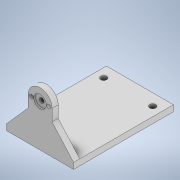
# Autodesk Inventor part: encoder_mount
Saved by Autodesk Inventor 2022 (Build 260153000, 153)
## iProperties
Created: 2021-12-21
Part Number: encoder_mount
Material: Generic
Document SubType Name: Modeling
Designer: Emazuddin Alif
Density: 1 g/cm^3
Appearance: Default
Author: Emazuddin Alif
Autodesk Inventor part; units mm, degrees
ref_plane "YZ Plane" through (0, 0, 0) normal (1, 0, 0) x (0, 1, 0)
ref_plane "XZ Plane" through (0, 0, 0) normal (0, 1, 0) x (-1, 0, 0)
ref_plane "XY Plane" through (0, 0, 0) normal (0, 0, 1) x (1, 0, 0)
sketch "Sketch1" plane through (0, 0, 0) normal (0, 0, 1) x (1, 0, 0)
  arc A0 (3.5804, 13.0349) -> (-21.4196, 13.0349) centre (-8.9196, 13.0349) ccw
  line L0 (-21.4196, 13.0349) -> (-21.4196, -24.5571)
  line L1 (-21.4196, -24.5571) -> (3.5804, -24.5571)
  line L2 (3.5804, 13.0349) -> (3.5804, -24.5571)
  circle A1 centre (-8.9196, 13.0349) radius 2.54
  point P0 (0, 0)
  dimension "d10" = 5.08
  dimension "d11" = 12.5
  dimension "d12" = 37.592
  constraints: 6 end point, 2 centre point, 2 perpendicular, 2 point on circle, 2 tangent, 1 coincident, 1 vertical
  measures "d10" diameter of A1
  measures "d11" radius of A0
  measures "d12" distance from line of L1 A0.centre
extrude "Extrusion1" add sketch "Sketch1" along normal blind 6.35
sketch "Sketch2" plane through (0, 0, 6.35) normal (0, 0, 1) x (1, 0, 0)
  circle A0 centre (-8.9196, 13.0349) radius 2.54 projected
  circle A1 centre (-8.9196, 13.0349) radius 6.5
  point P0 (0, 0)
  dimension "d9" = 13
  constraints: 1 centre point, 1 coincident
  measures "d9" diameter of A1
extrude "Extrusion2" cut sketch "Sketch2" against normal blind 1.778
sketch "Sketch4" plane through (-21.4196, -24.5571, 0) normal (0, -1, 0) x (1, 0, 0)
  line L0 (-22.425, 6.35) -> (47.425, 6.35)
  line L1 (47.425, 6.35) -> (47.425, -97.79)
  line L2 (47.425, -97.79) -> (-22.425, -97.79)
  line L3 (-22.425, -97.79) -> (-22.425, 6.35)
  line L4 (0, 0) -> (0, 6.35) projected
  line L5 (0, 6.35) -> (0, -15.1092)
  line L6 (12.5, -94.4689) -> (12.5, -35.8122)
  line L7 (0, 6.35) -> (25, 6.35) projected
  point P0 (21.4196, 0)
  dimension "d15" = 12.5
  dimension "d16" = 69.85
  dimension "d17" = 104.14
  constraints: 10 end point, 3 vertical, 2 horizontal, 1 parallel, 1 point on line, 4 other
  measures "d15" distance between parallel lines of L6 L5
  measures "d16" distance of L1.end L2.end
  measures "d17" distance of L2.end L3.end
extrude "Extrusion5" add sketch "Sketch4" along normal blind 6.35
sketch "Sketch5" plane through (0, 0, 6.35) normal (0, 0, 1) x (1, 0, 0)
  line L0 (-43.8446, -24.5571) -> (-43.8446, -30.9071) projected
  line L1 (-21.4196, -24.5571) -> (-43.8446, -24.5571) projected
  line L2 (-43.8446, -24.5571) -> (-21.4196, -24.5571)
  line L3 (-21.4196, -24.5571) -> (-21.4196, 0.8429)
  line L4 (-21.4196, 13.0349) -> (-21.4196, -24.5571) projected
  line L5 (-43.8446, -24.5571) -> (-21.4196, 0.8429)
  line L6 (26.0054, -24.5571) -> (3.5804, -24.5571) projected
  line L7 (26.0054, -24.5571) -> (3.5804, 0.8429)
  line L8 (3.5804, 0.8429) -> (3.5804, -24.5571)
  line L9 (3.5804, -24.5571) -> (26.0054, -24.5571)
  point P0 (0, 0)
  dimension "d20" = 25.4
  dimension "d21" = 25.4
  constraints: 12 end point, 2 perpendicular, 1 collinear, 1 point on line
  measures "d20" distance of L1.start L3.end
  measures "d21" distance of L7.end L6.end
extrude "Extrusion6" add sketch "Sketch5" against normal blind 6.35
sketch "Sketch6" plane through (0, 0, 0) normal (0, 0, -1) x (-1, 0, 0)
  circle A0 centre (8.9196, 13.0349) radius 2.54 projected
  line L0 (8.9196, 13.0349) -> (8.9196, 0.8013)
  circle A1 centre (17.9196, 13.0349) radius 2
  circle A2 centre (-0.0804, 13.0349) radius 2
  point P0 (0, 0)
  dimension "d24" = 18
  dimension "d25" = 4
  constraints: 2 centre point, 2 end point, 1 symmetric about line, 1 vertical, 1 other
  measures "d24" diameter of A1.centre L0
  measures "d25" diameter of A1
extrude "Extrusion7" cut sketch "Sketch6" against normal through all contours A1 | A2
sketch "Sketch7" plane through (-21.4196, -30.9071, 0) normal (0, -1, 0) x (1, 0, 0)
  circle A0 centre (-13.0588, -85.598) radius 3.175
  line L0 (12.5, -78.7871) -> (12.5, -99.3381)
  circle A1 centre (38.0588, -85.598) radius 3.175
  line L1 (47.425, 6.35) -> (-22.425, 6.35) projected
  point P0 (21.4196, 0)
  dimension "d28" = 6.35
  dimension "d29" = 51.1175
  dimension "d30" = 91.948
  constraints: 2 centre point, 2 end point, 1 symmetric about line, 1 vertical, 1 other
  measures "d28" diameter of A0
  measures "d29" diameter of A0.centre L0
  measures "d30" distance from line of L1 A0.centre
extrude "Extrusion8" cut sketch "Sketch7" against normal through all
body "Solid1"
